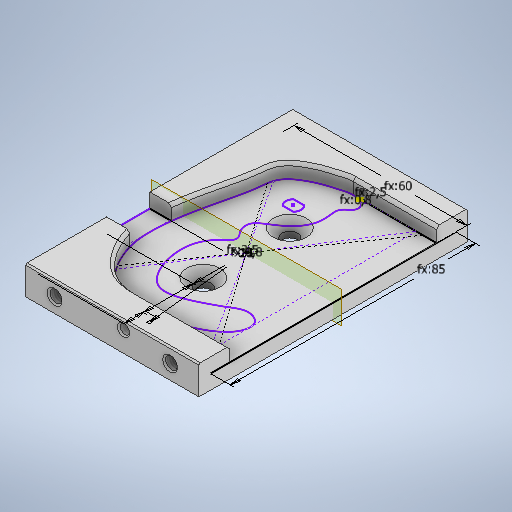
# Autodesk Inventor part: TS_V1_Fallmagazin_Wandung_int
Saved by Autodesk Inventor 2025.2 (Build 292293000, 293)
## iProperties
Created: 2025-06-10
Part Number: TS_V1_Fallmagazin_Wandung_int
Material: Generisch
Document SubType Name: Modeling
Designer: tino
Density: 1 g/cm^3
Appearance: Vorgabe
Author: tino
Autodesk Inventor part; units mm, degrees
ref_plane "YZ Plane" through (0, 0, 0) normal (1, 0, 0) x (0, 1, 0)
ref_plane "XY Plane" through (0, 0, 0) normal (0, 0, 1) x (1, 0, 0)
sketch "Skizze1" plane through (0, 0, 0) normal (0, 0, 1) x (1, 0, 0)
  arc A0 (-7.9107, 24.207) -> (-7.9109, 20.407) centre (-6.0635, 22.307) ccw
  line L0 (-7.9107, 24.207) -> (-4.2161, 24.2069)
  arc A1 (-4.2163, 20.4069) -> (-4.2161, 24.2069) centre (-6.0635, 22.307) ccw
  line L1 (-4.2163, 20.4069) -> (-7.9109, 20.407)
  spline S0 degree 3 poles (4.1682, 35.1897) (1.1905, 36.4598) (-2.2497, 35.1642) (-6.255, 34.1582) (-11.7361, 32.1479) (-17.2675, 27.437) (-17.3979, 22.2805) (-19.1794, 11.8373) (-24.2043, -4.2198) (-21.9122, -21.3619) (-15.7263, -32.1361) (-8.9601, -34.8731) (-7.7344, -35.2068) knots 0 0 0 0 0.05535 0.076528 0.211782 0.295547 0.382964 0.432922 0.754884 0.81234 0.967238 1 1 1 1
  spline S1 degree 3 poles (-7.7344, -35.2068) (-2.4391, -36.6482) (4.9342, -35.145) (14.3889, -31.3641) (20.2206, -28.2766) (23.0847, -23.1792) (23.281, -18.9959) (17.3062, -16.4997) (13.7398, -19.2937) (6.9074, -22.9332) (-1.1986, -27.1621) (-10.3055, -22.9326) (-14.0352, -10.4002) (-9.4599, -0.926) (-6.8334, 0.3153) (-5.9182, 2.0588) (-5.9367, 4.1791) (-8.2887, 5.2306) (-8.3642, 10.4373) (-1.0106, 14.1251) (4.0821, 20.0507) (3.0635, 26.3026) (2.9493, 28.6136) (3.7888, 29.834) (5.5778, 31.0924) (6.6132, 32.7745) (5.2458, 34.7086) (4.2656, 35.1481) (4.1682, 35.1897) knots 0 0 0 0 0.14153 0.17035 0.245987 0.25892 0.290227 0.326265 0.372233 0.38898 0.482096 0.508256 0.624416 0.647418 0.715274 0.72607 0.746892 0.801722 0.811885 0.848514 0.916356 0.943374 0.948219 0.962959 0.96651 0.98188 0.998188 1 1 1 1
  line L2 (-4.2163, 20.4069) -> (-7.9109, 20.407)
  arc A2 (-4.2163, 20.4069) -> (-4.2161, 24.2069) centre (-6.0635, 22.307) ccw
  line L3 (-7.9107, 24.207) -> (-4.2161, 24.2069)
  arc A3 (-7.9107, 24.207) -> (-7.9109, 20.407) centre (-6.0635, 22.307) ccw
  line L4 (-22.9949, 35.8296) -> (22.9949, 35.8296) construction
  line L5 (22.9949, 35.8296) -> (22.9949, -35.8296) construction
  line L6 (22.9949, -35.8296) -> (-22.9949, -35.8296) construction
  line L7 (-22.9949, -35.8296) -> (-22.9949, 35.8296) construction
  line L8 (-22.9949, 35.8296) -> (22.9949, -35.8296) construction
  line L9 (-22.9949, -35.8296) -> (22.9949, 35.8296) construction
  circle A4 centre (3.8745, -36.2796) radius 1.25 construction
  line L10 (1.2146, -35.8296) -> (11.5877, -35.8296) construction
  line L11 (3.8745, -36.2796) -> (3.8745, -35.0296) construction
  circle A5 centre (4.7955, 36.2796) radius 1.25 construction
  line L12 (4.7955, 36.2796) -> (4.7955, 35.0296) construction
  line L13 (3.124, 35.8296) -> (12.547, 35.8296) construction
  point P0 (0, 0)
  point P1 (0, 0)
  point P2 (0, 0)
  dimension "d88" = 2.5
  dimension "d91" = 2.5
  dimension "d89" = 0.8
  dimension "d92" = 0.8
  constraints: 28 end point, 8 point on circle, 4 centre point, 4 perpendicular, 3 vertical, 2 collinear, 2 horizontal, 2 midpoint, 2 vertical alignment, 1 coincident, 8 other
sketch "Skizze9" plane through (0, 0, 0) normal (0, 0, 1) x (1, 0, 0)
  line L0 (-30, 42.5) -> (30, 42.5)
  line L1 (30, 42.5) -> (30, -42.5)
  line L2 (30, -42.5) -> (-30, -42.5)
  line L3 (-30, -42.5) -> (-30, 42.5)
  line L4 (-30, 42.5) -> (30, -42.5) construction
  line L5 (30, 42.5) -> (-30, -42.5) construction
  line L6 (-2.7819, -35.8296) -> (30, -35.8296)
  line L7 (1.074, 35.8296) -> (30, 35.8296)
  line L8 (-30, -18.5) -> (-21.9819, -18.5)
  line L9 (-22.5463, -3.5) -> (-30, -3.5)
  line L10 (-30, -3.5) -> (-30, -18.5)
  spline S0 degree 3 poles (4.1682, 35.1897) (1.1905, 36.4598) (-2.2497, 35.1642) (-6.255, 34.1582) (-11.7361, 32.1479) (-17.2675, 27.437) (-17.3979, 22.2805) (-19.1794, 11.8373) (-24.2043, -4.2198) (-21.9122, -21.3619) (-15.7263, -32.1361) (-8.9601, -34.8731) (-7.7344, -35.2068) knots 0 0 0 0 0.05535 0.076528 0.211782 0.295547 0.382964 0.432922 0.754884 0.81234 0.967238 1 1 1 1
  spline S1 degree 3 poles (-7.7344, -35.2068) (-2.4391, -36.6482) (4.9342, -35.145) (14.3889, -31.3641) (20.2206, -28.2766) (23.0847, -23.1792) (23.281, -18.9959) (17.3062, -16.4997) (13.7398, -19.2937) (6.9074, -22.9332) (-1.1986, -27.1621) (-10.3055, -22.9326) (-14.0352, -10.4002) (-9.4599, -0.926) (-6.8334, 0.3153) (-5.9182, 2.0588) (-5.9367, 4.1791) (-8.2887, 5.2306) (-8.3642, 10.4373) (-1.0106, 14.1251) (4.0821, 20.0507) (3.0635, 26.3026) (2.9493, 28.6136) (3.7888, 29.834) (5.5778, 31.0924) (6.6132, 32.7745) (5.2458, 34.7086) (4.2656, 35.1481) (4.1682, 35.1897) knots 0 0 0 0 0.14153 0.17035 0.245987 0.25892 0.290227 0.326265 0.372233 0.38898 0.482096 0.508256 0.624416 0.647418 0.715274 0.72607 0.746892 0.801722 0.811885 0.848514 0.916356 0.943374 0.948219 0.962959 0.96651 0.98188 0.998188 1 1 1 1
  point P0 (0, 0)
  dimension "d68" = 60
  dimension "d69" = 85
  dimension "d75" = 15
  dimension "d76" = 24
  constraints: 22 end point, 4 horizontal, 3 parallel, 3 perpendicular, 3 point on line, 2 midpoint, 2 other
  measures "d68" distance of L0.start L0.end
  measures "d69" distance of L0.end L1.end
  measures "d75" distance between parallel lines of L9 L8
  measures "d76" distance between parallel lines of L2 L8
extrude "Extrusion3" add sketch "Skizze9" along normal blind 5 contours L0 L1 L7 S0 L9 L3 | L8 S0 S1 L6 L1 L2 L3
sketch "Skizze11" plane through (0, 0, 0) normal (0, 0, -1) x (-1, 0, 0)
  line L0 (30, -42.5) -> (-30, -42.5) projected
  line L1 (30, 42.5) -> (30, -42.5) projected
  line L2 (-30, -42.5) -> (30, -42.5)
  line L3 (30, -42.5) -> (30, 42.5)
  line L4 (30, 42.5) -> (-30, 42.5)
  line L5 (-30, 42.5) -> (-30, -42.5)
  point P0 (0, 0)
  constraints: 8 end point, 2 parallel, 1 horizontal, 1 perpendicular
extrude "Extrusion4" add sketch "Skizze11" along normal blind 1.5
chamfer "Fasen2" distance 1 angle 45 2 edges at (13.609, -35.8296, 5) (15.537, 35.8296, 5)
sketch "Skizze15" plane through (-30, 42.5, 5) normal (0, 1, 0) x (1, 0, 0)
  line L0 (60, 0) -> (0, 0) projected
  line L1 (0, 6.5) -> (60, 6.5) projected
  line L2 (60, 0) -> (0, 0)
  line L3 (0, 0) -> (0, 6.5)
  line L4 (0, 6.5) -> (60, 6.5)
  line L5 (60, 6.5) -> (60, 0)
  point P0 (30, 5)
  constraints: 8 end point, 2 parallel, 1 horizontal, 1 perpendicular
extrude "Extrusion6" add sketch "Skizze15" along normal blind 4
sketch "Skizze16" plane through (-30, -42.5, 5) normal (0, -1, 0) x (1, 0, 0)
  line L0 (0, -6.5) -> (0, 0) projected
  line L1 (60, -6.5) -> (0, -6.5) projected
  line L2 (0, 0) -> (60, 0)
  line L3 (60, 0) -> (60, -6.5)
  line L4 (60, -6.5) -> (0, -6.5)
  line L5 (0, -6.5) -> (0, 0)
  point P0 (30, -5)
  constraints: 8 end point, 2 parallel, 1 horizontal, 1 perpendicular
extrude "Extrusion7" add sketch "Skizze16" along normal blind 4
sketch "Skizze12" plane through (-2.7819, -35.8296, 0) normal (0, 1, 0) x (1, 0, 0)
  line L0 (5.4065, 0) -> (7.9065, 0) construction
  line L1 (32.7819, -4) -> (0, -4) projected
  point P0 (2.7819, 0)
  point P1 (6.6565, 0)
  point P2 (6.6565, 0)
  point P3 (6.6565, 0)
  point P4 (6.6565, -2)
  point P5 (6.6565, 0)
  dimension "d95" = 4
  dimension "d96" = 2
  constraints: 1 midpoint, 1 vertical alignment
  measures "d95" distance between parallel lines of L1 L0
  measures "d96" distance from line of L1 point (6.656, -2)
hole "Bohrung6" at (3.8745, -35.8296, 2) direction (0, -1, 0) diameter 3.242 end through all thread size "M4x0.7" class "6H" standard "ISO Metric profile"
sketch "Skizze13" plane through (1.074, 35.8296, 0) normal (0, -1, 0) x (1, 0, 0)
  line L0 (4.9715, 0) -> (2.4715, 0) construction
  line L1 (0, 0) -> (28.926, 0) projected
  line L2 (28.926, 5) -> (0, 5) projected
  line L3 (-31.074, -1.5) -> (28.926, -1.5) projected
  line L4 (0, 4) -> (28.926, 4) projected
  point P0 (-1.074, 0)
  point P1 (3.7215, 0)
  point P2 (3.7215, 0)
  point P3 (3.7215, 0)
  point P4 (3.7215, 2)
  dimension "d126" = 4
  dimension "d127" = 2
  constraints: 1 vertical alignment
  measures "d126" distance between parallel lines of L4 L1
  measures "d127" distance from line of L4 point (3.722, 2)
hole "Bohrung7" at (4.7955, 35.8296, 2) direction (0, 1, 0) diameter 3.242 end through all thread size "M4x0.7" class "6H" standard "ISO Metric profile"
sketch "Skizze17" plane through (0, 0, -1.5) normal (0, 0, -1) x (-1, 0, 0)
  line L0 (30, 46.5) -> (30, -46.5) projected
  line L1 (-30, 46.5) -> (30, 46.5) projected
  line L2 (-30, -46.5) -> (-30, 46.5) projected
  line L3 (30, -46.5) -> (-30, -46.5) projected
  point P0 (0, 0)
extrude "Extrusion8" add sketch "Skizze17" along normal blind 3.5
chamfer "Fasen4" distance 0.5 angle 45 4 edges at (3.8745, -46.5, 0.379) (4.7955, 46.5, 3.621) (0, 46.5, 5) (0, -46.5, 5)
sketch "Skizze20" plane through (0, 0, 0) normal (0, 0, 1) x (1, 0, 0)
  line L0 (-30, -46.5) -> (30, -46.5) projected
  line L1 (30, 35.8296) -> (30, -35.8296) projected
  point P0 (0, 0)
  point P1 (0, -15)
  point P2 (0, 0)
  point P3 (0, 15)
  dimension "d152" = 15
  dimension "d153" = 15
  constraints: 2 vertical alignment
  measures "d152" distance of point (0, -15) point (0, 0)
  measures "d153" distance of point (0, 15) point (0, 0)
hole "Bohrung10" at (0, -15, 0) at (0, 15, 0) direction (0, 0, -1) diameter 5.5 end through all countersink diameter 11.5 countersink angle 90
sketch "Skizze21" plane through (-30, -46.5, 5) normal (0, -1, 0) x (1, 0, 0)
  line L0 (60, -10) -> (0, -10) projected
  line L1 (60, 0) -> (0, 0) projected
  line L2 (60, -0.5) -> (60, -10) projected
  line L3 (0, -0.5) -> (0, -10) projected
  point P0 (30, -5)
  point P1 (10, -5)
  point P2 (50, -5)
  point P3 (60, -5.25)
  dimension "d161" = 10
  dimension "d162" = 5
  dimension "d163" = 60
  dimension "d164" = 10
  dimension "d165" = 10
  constraints: 1 horizontal alignment, 1 midpoint
  measures "d161" distance between parallel lines of L0 L1
  measures "d162" distance from line of L1 point (10, -5)
  measures "d163" distance between parallel lines of L2 L3
  measures "d164" distance from line of L3 point (10, -5)
  measures "d165" horizontal distance of point (60, -5.25) point (50, -5)
hole "Bohrung11" at (20, -46.5, 0) at (-20, -46.5, 0) direction (0, 1, 0) diameter 4.134 depth 6 tip angle 118 thread size "M5x0.8" class "6H" standard "ISO Metric profile"
chamfer "Fasen5" distance 0.5 angle 45 2 edges at (-20, -46.5, 2.067) (20, -46.5, 2.067)
mirror "Spiegeln4" about plane through (0, 0, 0) normal (0, 1, 0) of "Bohrung11"
chamfer "Fasen6" distance 0.5 angle 45 2 edges at (20, 46.5, 2.067) (-20, 46.5, 2.067)
equation "\"d88\" = Kugeldurchmesser"
equation "\"d91\" = Kugeldurchmesser"
equation "\"d89\" = Kugelhoehe"
equation "\"d92\" = Kugelhoehe"
equation "\"d68\" = Breite_innen"
equation "\"d69\" = Laenge_innen"
equation "\"d96\" = 0.5 * d95"
equation "\"d127\" = 0.5 * d126"
equation "\"d152\" = Anbindung_Kolben"
equation "\"d153\" = d152"
equation "\"d162\" = 0.5 * d161"
equation "\"Breite_innen\" = 60"
equation "\"Laenge_innen\" = 85"
equation "\"Laenge_aussen\" = Laenge_innen + 2 * Wanddicke"
equation "\"Absatz\" = 2"
equation "\"Kugeldurchmesser\" = 2.5"
equation "\"Kugelhoehe\" = 0.8"
equation "\"Anbindung_Kolben\" = 15"
equation "\"Wanddicke\" = 10"
